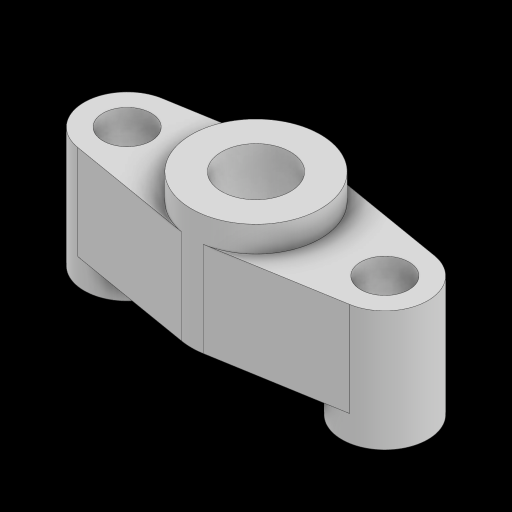
# Autodesk Inventor part: 250_CameraMount
Saved by Autodesk Inventor 2024 (Build 280153000, 153)
## iProperties
Created: 2023-07-21
Part Number: 250_CameraMount
Material: Generisch
Document SubType Name: Modeling
Designer: Philipp
Density: 1 g/cm^3
Appearance: Vorgabe
Author: Philipp
Autodesk Inventor part; units mm, degrees
ref_plane "YZ Plane" through (0, 0, 0) normal (1, 0, 0) x (0, 1, 0)
ref_plane "XZ Plane" through (0, 0, 0) normal (0, 1, 0) x (-1, 0, 0)
sketch "Skizze1" plane through (0, 0, 0) normal (0, 0, 1) x (1, 0, 0)
  circle A0 centre (0, 0) radius 7.5
  circle A1 centre (0, 0) radius 4
  dimension "d0" = 15
  dimension "d3" = 8
  constraints: 2 centre point, 2 coincident
  measures "d0" diameter of A0
  measures "d3" diameter of A1
extrude "Extrusion1" add sketch "Skizze1" against normal blind 14
ref_plane "Arbeitsebene1" through (0, 0, -3) normal (0, 0, 1) x (1, 0, 0)
sketch "Skizze2" plane through (0, 0, -3) normal (0, 0, 1) x (1, 0, 0)
  circle A0 centre (-15, 0) radius 5
  circle A1 centre (15, 0) radius 5
  circle A2 centre (-15, 0) radius 2.8
  circle A3 centre (15, 0) radius 2.8
  point P0 (0, 0)
  dimension "d5" = 10
  dimension "d6" = 10
  dimension "d7" = 15
  dimension "d8" = 15
  dimension "d9" = 5.6
  dimension "d10" = 5.6
  constraints: 4 centre point, 2 coincident
  measures "d5" diameter of A0
  measures "d6" diameter of A1
  measures "d7" distance of point (0, 0) A0.centre
  measures "d8" distance of A1.centre point (0, 0)
  measures "d9" diameter of A2
  measures "d10" diameter of A3
extrude "Extrusion2" add sketch "Skizze2" against normal blind 14
sketch "Skizze3" plane through (-15, 0, -3) normal (0, 0, 1) x (1, 0, 0)
  circle A0 centre (0, 0) radius 5 projected
  circle A1 centre (0, 0) radius 2.8 projected
  circle A2 centre (15, 0) radius 7.5 projected
  circle A3 centre (15, 0) radius 4 projected
  circle A4 centre (30, 0) radius 5 projected
  circle A5 centre (30, 0) radius 2.8 projected
  circle A6 centre (15, 0) radius 7.5 projected
  line L0 (-5.1094, 4.2073) -> (15, 7.6064)
  line L1 (15, 7.6064) -> (38.7432, 3.5931)
  circle A7 centre (30, 0) radius 5 projected
  line L2 (-7.8587, -3.7426) -> (15, -7.6064)
  line L3 (15, -7.6064) -> (39.1845, -3.5185)
  point P0 (16.25, -7.3951)
  point P1 (30.8333, -4.9301)
  point P2 (30.8333, 4.9301)
  point P3 (16.25, 7.3951)
  point P4 (-0.8333, -4.9301)
  point P5 (13.75, -7.3951)
  point P6 (13.75, 7.3951)
  point P7 (-0.8333, 4.9301)
  constraints: 8 end point, 8 tangent
extrude "Extrusion3" add sketch "Skizze3" against normal blind 11 contours A0 L0 A2 L2 | L1 A4 L3 A2
